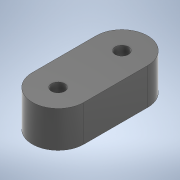
# Autodesk Inventor part: 08-02-01-009_fixPCBSpacer
Saved by Autodesk Inventor 2020 (Build 240168000, 168)
## iProperties
Created: 2021-07-28
Part Number: 08-02-01-009_fixPCBSpacer
Material: ABS-Kunststoff(1)
Document SubType Name: Modeling
Designer: Eric
Density: 1.06 g/cm^3
Appearance: Glatt - Weiß(1)
Author: Eric
## iProperties of the stored document _3D-Druck.ipt
Created: 2021-08-26
Part Number: _3D-Druck
Material: Generisch
Document SubType Name: Modeling
Designer: Eric
Density: 1 g/cm^3
Appearance: Vorgabe
Author: Eric
Autodesk Inventor part; units mm, degrees
ref_plane "YZ Plane" through (0, 0, 0) normal (1, 0, 0) x (0, 1, 0)
ref_plane "XZ Plane" through (0, 0, 0) normal (0, 1, 0) x (-1, 0, 0)
ref_plane "XY Plane" through (0, 0, 0) normal (0, 0, 1) x (1, 0, 0)
sketch "Skizze1" plane through (0, 0, 0) normal (0, 1, 0) x (-1, 0, 0)
  circle A0 centre (0, 5) radius 1.05
  circle A1 centre (0, -5) radius 1.05
  line L0 (0, 5) -> (0, -5) construction
  line L1 (0, 5) -> (0, -5) construction
  line L2 (-4.05, 5) -> (-4.05, -5)
  line L3 (4.05, -5) -> (4.05, 5)
  arc A2 (4.05, 5) -> (-4.05, 5) centre (0, 5) ccw
  arc A3 (-4.05, -5) -> (4.05, -5) centre (0, -5) ccw
  point P0 (0, 0)
  point P1 (0, 0)
  point P2 (0, 0)
  dimension "d0" = 2.1
  dimension "d1" = 3
  dimension "d2" = 10
  constraints: 10 end point, 4 centre point, 4 point on circle, 4 tangent, 2 equal length, 2 midpoint, 1 coincident, 1 equal radius, 1 vertical
  measures "d0" diameter of A0
  measures "d1" radial gap between concentric circles of A2 A0
  measures "d2" distance of L0.end L0.start
extrude "Extrusion1" add sketch "Skizze1" along normal blind 5.7
